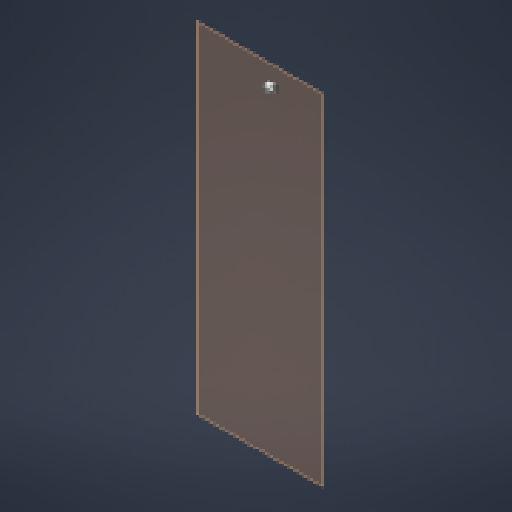
# Autodesk Inventor part: BracketSpacer
Saved by Autodesk Inventor 2026.2 (Build 302298000, 298)
## iProperties
Created: 2026-03-15
Part Number: BracketSpacer
Material: Generic
Document SubType Name: Modeling
Designer: brand
Density: 1 g/cm^3
Appearance: Default
Author: brand
Autodesk Inventor part; units mm, degrees
ref_plane "YZ Plane" through (0, 0, 0) normal (1, 0, 0) x (0, 1, 0)
ref_plane "XZ Plane" through (0, 0, 0) normal (0, 1, 0) x (-1, 0, 0)
ref_plane "XY Plane" through (0, 0, 0) normal (0, 0, 1) x (1, 0, 0)
ref_plane "Work Plane1" through (0, 0, 0) normal (0, 0, 1) x (1, 0, 0)
sketch "Sketch1" plane through (0, 0, 0) normal (0, 0, 1) x (1, 0, 0)
  circle A0 centre (173.6996, 946.853) radius 5.5 projected
  circle A1 centre (152.6996, 946.853) radius 5.5 projected
  line L0 (454.025, 962.025) -> (-295.275, 962.025) projected
  line L1 (-295.275, 962.025) -> (-295.275, -1057.275) projected
  line L2 (-295.275, -1057.275) -> (454.025, -1057.275) projected
  line L3 (454.025, -1057.275) -> (454.025, 962.025) projected
  circle A2 centre (396.1257, -28.5814) radius 31.4325 projected
  line L4 (182.6996, 962.025) -> (142.6996, 962.025)
  line L5 (142.6996, 962.025) -> (142.6996, 929.853)
  line L6 (142.6996, 929.853) -> (182.6996, 929.853)
  line L7 (182.6996, 929.853) -> (182.6996, 962.025)
  line L8 (195.3996, 917.153) -> (129.9996, 917.153)
  line L9 (129.9996, 917.153) -> (129.9996, 974.725)
  line L10 (129.9996, 974.725) -> (195.3996, 974.725)
  line L11 (195.3996, 974.725) -> (195.3996, 917.153)
  point P0 (0, 0)
  point P1 (182.6996, 963.853)
  point P2 (129.9996, 962.025)
  point P3 (195.3996, 962.025)
  dimension "d0" = 12.7
  constraints: 16 end point, 4 parallel, 2 perpendicular, 2 point on line, 1 horizontal, 5 other
  measures "d0" distance between parallel lines of L6 L8
extrude "Extrusion1" add sketch "Sketch1" along normal blind 49.5554 contours L7 L6 L5 L0
extrude "Extrusion2" add sketch "Sketch1" along normal blind 6.35 contours L0 L11 L8 L9 L5 L6 L7
fillet "Fillet1" radius 3.175 5 edges at (182.6996, 945.939, 6.35) (162.6996, 929.853, 6.35) (142.6996, 945.939, 6.35) (142.6996, 929.853, 27.9527) (182.6996, 929.853, 27.9527)
fillet "Fillet2" radius 3.175 2 edges at (129.9996, 962.025, 3.175) (195.3996, 962.025, 3.175)
fillet "Fillet3" radius 15.875 2 edges at (129.9996, 917.153, 3.175) (195.3996, 917.153, 3.175)
body "Solid1"
